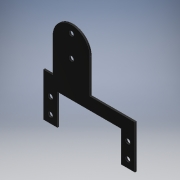
# Autodesk Inventor part: Wrist Servo Plate
Saved by Autodesk Inventor 2017 (Build 210142000, 142)
## iProperties
Created: 2018-10-18
Part Number: Wrist Servo Plate
Material: Generic
Document SubType Name: Modeling
Designer: Cameron
Density: 1 g/cm^3
Appearance: Glossy - Black
Author: Cameron
Autodesk Inventor part; units mm, degrees
ref_plane "YZ Plane" through (0, 0, 0) normal (1, 0, 0) x (0, 1, 0)
ref_plane "XZ Plane" through (0, 0, 0) normal (0, 1, 0) x (-1, 0, 0)
ref_plane "XY Plane" through (0, 0, 0) normal (0, 0, 1) x (1, 0, 0)
sketch "Sketch1" plane through (0, 0, 0) normal (0, 1, 0) x (-1, 0, 0)
  line L0 (12, 0) -> (12, 0)
  line L1 (24, -12) -> (24, -34)
  line L2 (0, -34) -> (0, -12)
  arc A0 (24, -12) -> (12, 0) centre (12, -12) ccw
  arc A1 (12, 0) -> (0, -12) centre (12, -12) ccw
  line L3 (0, -34) -> (-29, -34)
  line L4 (-29, -34) -> (-29, -62)
  line L5 (-29, -62) -> (-20, -62)
  line L6 (-20, -62) -> (-20, -42)
  line L7 (-20, -42) -> (21, -42)
  line L8 (21, -42) -> (21, -62)
  line L9 (21, -62) -> (30, -62)
  line L10 (30, -62) -> (30, -34)
  line L11 (30, -34) -> (24, -34)
  line L12 (25.5, -62) -> (25.5, -57)
  line L13 (25.5, -57) -> (25.5, -47)
  circle A2 centre (25.5, -57) radius 1.5
  circle A3 centre (25.5, -47) radius 1.5
  line L14 (25.5, -57) -> (-24.5, -57)
  line L15 (-24.5, -57) -> (-24.5, -47)
  circle A4 centre (-24.5, -47) radius 1.5
  circle A5 centre (-24.5, -57) radius 1.5
  point P0 (0, 0)
  point P1 (24, 0)
  dimension "d0" = 24
  dimension "d1" = 34
  dimension "d2" = 12
  dimension "d3" = 29
  dimension "d4" = 28
  dimension "d5" = 9
  dimension "d6" = 20
  dimension "d7" = 41
  dimension "d8" = 9
  dimension "d9" = 5
  dimension "d10" = 10
  dimension "d11" = 3
  dimension "d12" = 3
  dimension "d13" = 3
  dimension "d14" = 3
  constraints: 32 end point, 9 perpendicular, 8 point on line, 6 centre point, 4 coincident, 4 point on circle, 4 tangent, 3 horizontal, 1 concentric, 1 midpoint, 1 parallel, 1 vertical
  measures "d0" distance of L1.end L2.start
  measures "d1" distance of point (24, 0) L1.end
  measures "d2" radius of A0
  measures "d3" distance of L2.start L3.end
  measures "d4" distance of L3.end L4.end
  measures "d5" distance of L4.end L5.end
  measures "d6" distance of L5.end L6.end
  measures "d7" distance of L6.end L7.end
  measures "d8" distance of L8.end L9.end
  measures "d9" distance of L12.start L12.end
  measures "d10" distance of L12.end L13.end
  measures "d11" diameter of A2
  measures "d12" diameter of A3
  measures "d13" diameter of A4
  measures "d14" diameter of A5
extrude "Extrusion1" add sketch "Sketch1" along normal blind 1 contours L1 L11 L10 L9 L12 A2 L14 L8 L7 L6 L5 L4 L3 L2 A1 A0 | L9 L8 L14 A2 L12
sketch "Sketch2" plane through (0, 1, 0) normal (0, 1, 0) x (1, 0, 0)
  arc A0 (-24, 12) -> (0, 12) centre (-12, 12) ccw projected
  circle A1 centre (-25.5, 57) radius 1.5 projected
  circle A2 centre (-25.5, 47) radius 1.5 projected
  line L0 (-25.5, 57) -> (-25.5, 47)
  line L1 (-12, 12) -> (-12, 19)
  line L2 (-12, 19) -> (-12, 5)
  circle A3 centre (-12, 5) radius 1.5
  circle A4 centre (-12, 19) radius 1.5
  point P0 (0, 0)
  dimension "d17" = 7
  dimension "d18" = 14
  dimension "d19" = 3
  dimension "d20" = 3
  constraints: 6 end point, 2 centre point, 2 coincident, 2 vertical, 1 point on line
  measures "d17" distance of L1.start L1.end
  measures "d18" distance of L1.end L2.end
  measures "d19" diameter of A3
  measures "d20" diameter of A4
extrude "Extrusion2" cut sketch "Sketch2" against normal blind 1 contours A4 | A3
body "Solid1"
